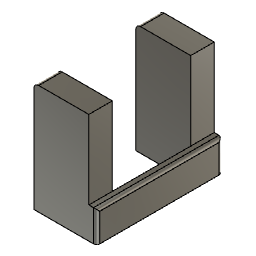
Z-AdjustBlock (Autodesk Fusion 360 design; units mm, degrees)
Autodesk Fusion 360 part; units mm, degrees
sketch "Sketch1" plane through (0, 0, 0) normal (0, 0, 1) x (1, 0, 0) in component "Spacer"
  line L0 (0, 0) -> (35, 0)
  line L1 (35, 0) -> (35, 15)
  line L2 (35, 15) -> (0, 15)
  line L3 (0, 15) -> (0, 0)
  line L4 (0, 65) -> (35, 65)
  line L5 (35, 65) -> (35, 80)
  line L6 (35, 80) -> (0, 80)
  line L7 (0, 80) -> (0, 65)
  line L8 (35, 0) -> (40, 0)
  line L9 (40, 0) -> (40, 80)
  line L10 (40, 80) -> (35, 80)
  line L11 (35, 80) -> (35, 0)
  dimension "d1" = 35
  dimension "d2" = 15
  dimension "d3" = 35
  dimension "d4" = 15
  dimension "d5" = 50
  dimension "d6" = 35
  dimension "d7" = 5
  dimension "d8" = 80
  constraint horizontal L0
  constraint vertical L1
  constraint horizontal L2
  constraint vertical L3
  constraint coincident L0.start L3.end
  constraint horizontal L4
  constraint vertical L5
  constraint horizontal L6
  constraint vertical L7
  constraint horizontal L8
  constraint vertical L9
  constraint horizontal L10
  constraint vertical L11
  measures "d1" distance of L0.start L0.end
  measures "d2" distance of L0.start L2.end
  measures "d3" distance of L4.start L4.end
  measures "d4" distance of L4.start L6.end
  measures "d5" distance of L2 L4
  measures "d6" distance of L3 L5
  measures "d7" distance of L5 L9
  measures "d8" distance of L0.start L10
extrude "Extrude1" add sketch "Sketch1" along normal blind 70 contours L0 L1 L2 L3 L11 | L4 L5 L6 L7 L11 makes body 1 at (23.3333, 15, 46.6667) makes body 2 at (11.6667, 65, 46.6667) in component "Spacer"
extrude "Extrude2" add sketch "Sketch1" along normal blind 20 contours L1 L5 L8 L9 L10 L11 bodies 1 2 in component "Spacer"
fillet "Fillet1" radius 2 3 edges at (40, 40, 20) (40, 0, 10) (40, 80, 10) on bodies 1 in component "Spacer"
fillet "Fillet2" radius 3 2 edges at (0, 72.5, 70) (0, 7.5, 70) on bodies 1 in component "Spacer"
component "Spacer" placed x (1, 0, 0) y (0, 1, 0) z (0, 0, 1) at (0, 0, 0)
